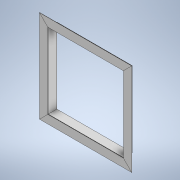
# Autodesk Inventor part: Test Section Frame
Saved by Autodesk Inventor 2022 (Build 260153000, 153)
## iProperties
Created: 2022-03-07
Part Number: Test Section Frame
Material: Generic
Document SubType Name: Modeling
Designer: calvi
Density: 1 g/cm^3
Appearance: Default
Author: calvi
Autodesk Inventor part; units mm, degrees
ref_plane "YZ Plane" through (0, 0, 0) normal (1, 0, 0) x (0, 1, 0)
ref_plane "XZ Plane" through (0, 0, 0) normal (0, 1, 0) x (-1, 0, 0)
ref_plane "XY Plane" through (0, 0, 0) normal (0, 0, 1) x (1, 0, 0)
sketch "Sketch1" plane through (0, 0, 0) normal (0, 0, 1) x (1, 0, 0)
  line L0 (-221.75, -221.75) -> (221.75, -221.75)
  line L1 (221.75, -221.75) -> (221.75, 221.75)
  line L2 (221.75, 221.75) -> (-221.75, 221.75)
  line L3 (-221.75, 221.75) -> (-221.75, -221.75)
  line L4 (-221.75, -221.75) -> (221.75, 221.75) construction
  line L5 (221.75, -221.75) -> (-221.75, 221.75) construction
  line L6 (-223.25, 223.25) -> (223.25, 223.25)
  line L7 (223.25, 223.25) -> (223.25, -223.25)
  line L8 (223.25, -223.25) -> (-223.25, -223.25)
  line L9 (-223.25, -223.25) -> (-223.25, 223.25)
  point P0 (0, 0)
  dimension "d0" = 443.5
  dimension "d1" = 443.5
  dimension "d2" = 1.5
  constraints: 20 end point, 4 parallel, 2 midpoint, 2 perpendicular, 1 horizontal, 3 other
  measures "d0" distance of L2.end L1.end
  measures "d1" distance of L1.end L0.end
  measures "d2" distance between parallel lines of L2 L6
extrude "Extrusion1" add sketch "Sketch1" along normal blind 50.8
sketch "Sketch2" plane through (0, 0, 50.8) normal (0, 0, 1) x (1, 0, 0)
  line L0 (272.55, -272.55) -> (-272.55, -272.55)
  line L1 (-272.55, -272.55) -> (-272.55, 272.55)
  line L2 (-272.55, 272.55) -> (272.55, 272.55)
  line L3 (272.55, 272.55) -> (272.55, -272.55)
  line L4 (272.55, -272.55) -> (-272.55, 272.55) construction
  line L5 (-272.55, -272.55) -> (272.55, 272.55) construction
  line L6 (223.25, 223.25) -> (-223.25, 223.25) projected
  line L7 (-272.55, 272.55) -> (-223.25, 223.25)
  line L8 (-223.25, 223.25) -> (-223.25, -223.25) projected
  line L9 (-272.55, -272.55) -> (-223.25, -223.25)
  line L10 (-223.25, -223.25) -> (223.25, -223.25) projected
  line L11 (272.55, -272.55) -> (223.25, -223.25)
  line L12 (272.55, 272.55) -> (223.25, 223.25)
  line L13 (223.25, -223.25) -> (223.25, 223.25) projected
  point P0 (0, 0)
  dimension "d5" = 545.1
  dimension "d6" = 545.1
  constraints: 20 end point, 2 midpoint, 2 parallel, 1 horizontal, 1 perpendicular
  measures "d5" distance of L1.end L2.end
  measures "d6" distance of L0.end L1.end
extrude "Extrusion2" add sketch "Sketch2" along normal blind 1.5 separate body contours L12 L6 L7 L2
extrude "Extrusion3" add sketch "Sketch2" along normal blind 1.5 separate body contours L11 L13 L12 L3
extrude "Extrusion4" add sketch "Sketch2" along normal blind 1.5 separate body contours L0 L9 L10 L11
extrude "Extrusion5" add sketch "Sketch2" along normal blind 1.5 separate body contours L1 L7 L8 L9
sketch "Sketch3" plane through (0, 0, 0) normal (0, 0, -1) x (-1, 0, 0)
  line L0 (-223.25, 223.25) -> (223.25, 223.25) projected
  line L1 (-223.25, -223.25) -> (-223.25, 223.25) projected
  line L2 (223.25, 223.25) -> (223.25, -223.25) projected
  line L3 (223.25, -223.25) -> (-223.25, -223.25) projected
  point P0 (0, 0)
body "Solid1"
body "Solid2"
body "Solid3"
body "Solid4"
body "Solid5"
